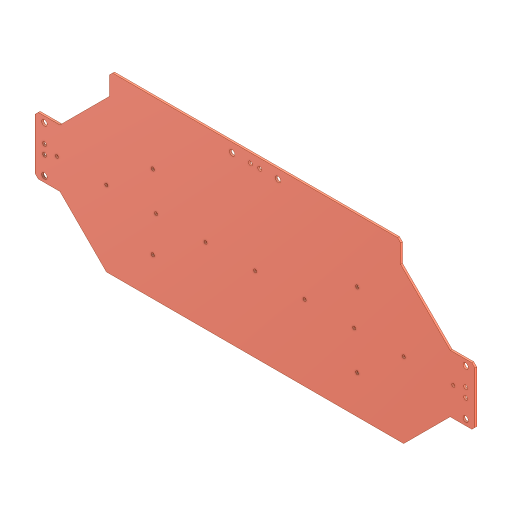
# Autodesk Inventor part: enc - FrontPanel Oben V2
Saved by Autodesk Inventor 2023.2 (Build 272271000, 271)
## iProperties
Created: 2023-12-14
Part Number: enc - FrontPanel Oben V2
Material: Generisch
Document SubType Name: Modeling
Designer: Nils Bade
Density: 1 g/cm^3
Appearance: RAL2008 Acryl
Description: Fertigung
Auf Bestellliste: True
Author: Nils Bade
Autodesk Inventor part; units mm, degrees
ref_plane "YZ Plane" through (0, 0, 0) normal (1, 0, 0) x (0, 1, 0)
ref_plane "XZ Plane" through (0, 0, 0) normal (0, 1, 0) x (-1, 0, 0)
ref_plane "XY Plane" through (0, 0, 0) normal (0, 0, 1) x (1, 0, 0)
sketch "Skizze1" plane through (0, 0, 0) normal (0, 0, 1) x (1, 0, 0)
  line L0 (-355, 166.5) -> (355, 166.5)
  line L1 (355, 166.5) -> (355, -166.5)
  line L2 (355, -166.5) -> (-355, -166.5)
  line L3 (-355, -166.5) -> (-355, 166.5)
  line L4 (-355, 166.5) -> (355, -166.5) construction
  line L5 (355, 166.5) -> (-355, -166.5) construction
  line L6 (-315, 126.5) -> (315, 126.5)
  line L7 (315, 126.5) -> (315, -126.5)
  line L8 (315, -126.5) -> (-315, -126.5)
  line L9 (-315, -126.5) -> (-315, 126.5)
  line L10 (0, 233.1) -> (0, -233.1) construction
  line L11 (-355, 46.5) -> (-315, 46.5)
  line L12 (-315, 46.5) -> (-235, 126.5)
  line L13 (-235, 126.5) -> (-235, 166.5)
  line L14 (-355, -46.5) -> (-315, -46.5)
  line L15 (-315, -46.5) -> (-235, -126.5)
  line L16 (-235, -126.5) -> (-235, -166.5)
  line L17 (355, 46.5) -> (315, 46.5)
  line L18 (315, 46.5) -> (235, 126.5)
  line L19 (235, 126.5) -> (235, 163.7426)
  line L20 (355, -46.5) -> (315, -46.5)
  line L21 (315, -46.5) -> (235, -126.5)
  line L22 (350, 161.5) -> (-350, 161.5)
  line L23 (-350, 161.5) -> (-350, -161.5)
  line L24 (-350, -161.5) -> (350, -161.5)
  line L25 (350, -161.5) -> (350, 161.5)
  circle A0 centre (-165, -60) radius 2.75
  line L26 (-153.5, -54) -> (-176.5, -54) construction
  line L27 (-176.5, -54) -> (-176.5, 54) construction
  line L28 (-176.5, 54) -> (-153.5, 54) construction
  line L29 (-153.5, 54) -> (-153.5, -54) construction
  line L30 (-153.5, -54) -> (-176.5, 54) construction
  line L31 (-176.5, -54) -> (-153.5, 54) construction
  line L32 (-497, 0) -> (497, 0) construction
  line L33 (-165, -54) -> (-165, 54) construction
  circle A1 centre (-165, 60) radius 2.75
  line L34 (176.5, 54) -> (153.5, 54) construction
  line L35 (153.5, 54) -> (153.5, -54) construction
  circle A2 centre (165, -60) radius 2.75
  line L36 (153.5, -54) -> (176.5, -54) construction
  line L37 (176.5, -54) -> (176.5, 54) construction
  circle A3 centre (165, 60) radius 2.75
  line L38 (-348, -45) -> (-332, -45) construction
  line L39 (-332, -45) -> (-332, 45) construction
  line L40 (-332, 45) -> (-348, 45) construction
  line L41 (-348, 45) -> (-348, -45) construction
  line L42 (-348, -45) -> (-332, 45) construction
  line L43 (-332, -45) -> (-348, 45) construction
  circle A4 centre (-340, -7.5) radius 3.25
  circle A5 centre (-340, -37) radius 4.5
  line L44 (-332, 0) -> (-348, 0) construction
  line L45 (-340, -45) -> (-340, 45) construction
  circle A6 centre (-340, 37) radius 4.5
  circle A7 centre (-340, 7.5) radius 3.25
  line L46 (-47.5, 154.5) -> (47.5, 154.5) construction
  line L47 (47.5, 154.5) -> (47.5, 138.5) construction
  line L48 (47.5, 138.5) -> (-47.5, 138.5) construction
  line L49 (-47.5, 138.5) -> (-47.5, 154.5) construction
  line L50 (-47.5, 154.5) -> (47.5, 138.5) construction
  line L51 (47.5, 154.5) -> (-47.5, 138.5) construction
  line L52 (-47.5, 146.5) -> (47.5, 146.5) construction
  circle A8 centre (-7.5, 146.5) radius 3.25
  circle A9 centre (-37, 146.5) radius 4.5
  circle A10 centre (7.5, 146.5) radius 3.25
  circle A11 centre (37, 146.5) radius 4.5
  circle A12 centre (340, -37) radius 4.5
  circle A13 centre (340, -7.5) radius 3.25
  circle A14 centre (340, 7.5) radius 3.25
  circle A15 centre (340, 37) radius 4.5
  circle A16 centre (0, 0) radius 2.5
  circle A17 centre (80, 0) radius 2.5
  circle A18 centre (160, 0) radius 2.5
  circle A19 centre (240, 0) radius 2.5
  circle A20 centre (320, 0) radius 2.5
  circle A21 centre (-80, 0) radius 2.5
  circle A22 centre (-160, 0) radius 2.5
  circle A23 centre (-240, 0) radius 2.5
  circle A24 centre (-320, 0) radius 2.5
  line L53 (-240, -121.5) -> (240, -121.5)
  line L54 (235, -126.5) -> (235, -166.5)
  point P0 (-235, 163.7426)
  point P1 (235, 161.5)
  point P2 (-235, 161.5)
  point P3 (-350, 46.5)
  point P4 (-350, -46.5)
  point P5 (-235, -126.5)
  point P6 (235, -126.5)
  point P7 (350, -46.5)
  point P8 (350, 46.5)
  point P9 (-165, 0)
  point P10 (-340, 0)
  point P11 (0, 146.5)
  point P12 (355, 46.5)
  dimension "d0" = 710
  dimension "d1" = 333
  dimension "d2" = 40
  dimension "d13" = 5
  dimension "d16" = 5.5
  dimension "d17" = 23
  dimension "d18" = 108
  dimension "d22" = 60
  dimension "d24" = 190
  dimension "d25" = 16
  dimension "d26" = 90
  dimension "d27" = 6.5
  dimension "d28" = 9
  dimension "d29" = 7.5
  dimension "d30" = 37
  dimension "d33" = 15
  dimension "d34" = 95
  dimension "d35" = 16
  dimension "d36" = 20
  dimension "d37" = 6.5
  dimension "d38" = 9
  dimension "d39" = 7.5
  dimension "d40" = 37
  dimension "d41" = 5
  dimension "d52" = 80
  dimension "d59" = 80
  dimension "d64" = 5
  dimension "d68" = 120
  dimension "d69" = 120
  dimension "d70" = 120
  dimension "d72" = 120
  dimension "d73" = 45
  dimension "d74" = 45
  constraints: 106 end point, 25 centre point, 23 symmetric about line, 16 midpoint, 16 point on line, 12 parallel, 8 perpendicular, 6 horizontal, 1 coincident, 1 vertical, 33 other
  measures "d0" distance of L0.start L0.end
  measures "d1" distance of L2.end L0.start
  measures "d2" distance between parallel lines of L3 L9
  measures "d13" distance between parallel lines of L0 L22
  measures "d16" diameter of A0
  measures "d17" distance of L28.start L28.end
  measures "d18" distance of L26.end L28.start
  measures "d22" distance from line of L32 A0.centre
  measures "d24" distance between parallel lines of L3 L33
  measures "d25" distance of L41.start L42.end
  measures "d26" distance of L42.end L38.end
  measures "d27" diameter of A4
  measures "d28" diameter of A5
  measures "d29" distance from line of L44 A4.centre
  measures "d30" distance from line of A5.centre L44
  measures "d33" distance between parallel lines of L3 L45
  measures "d34" distance of L47.end L48.end
  measures "d35" distance of L46.end L47.end
  measures "d36" distance between parallel lines of L0 L52
  measures "d37" diameter of A8
  measures "d38" diameter of A9
  measures "d39" distance from line of L10 A8.centre
  measures "d40" distance from line of L10 A9.centre
  measures "d41" diameter of A16
  measures "d52" distance of A16.centre A17.centre
  measures "d59" distance of A16.centre A21.centre
  measures "d64" distance between parallel lines of L8 L53
  measures "d68" distance between parallel lines of L0 L11
  measures "d69" distance between parallel lines of L3 L13
  measures "d70" distance between parallel lines of L2 L14
  measures "d72" distance between parallel lines of L3 L16
  measures "d73" angle of L3 L12
  measures "d74" angle of L2 L15
extrude "Extrusion1" add sketch "Skizze1" along normal blind 3 contours L11 L23 L14 L3 | L22 L19 L6 L13 | L11 L9 L14 L23 | L1 L20 L25 L17 | L6 L18 L7 L21 L53 L15 L9 L12 | L25 L20 L7 L17
chamfer "Fase-5mm" distance 5 angle 45 6 edges at (355, 46.5, 1.5) (355, -46.5, 1.5) (-355, -46.5, 1.5) (-355, 46.5, 1.5) (-235, 161.5, 1.5) (235, 161.5, 1.5)
equation "\"d37\" = d27"
equation "\"d38\" = d28"
equation "\"d39\" = d29"
equation "\"d40\" = d30"
equation "\"d59\" = d52"
